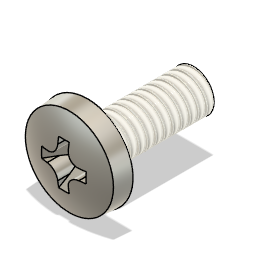
5e5ee204-5b50-4668-98c5-09c78f3fccee (Autodesk Fusion 360 design; units mm, degrees)
description: Parafuso de cabeça abaulada JIS B 1111 - M2x5
part number: BHS JIS B 1111 - M2x5 Aço 4.6 Liso
Autodesk Fusion 360 part; units mm, degrees
sketch "Sketch1" plane through (0, 0, 0) normal (0, 1, 0) x (1, 0, 0)
  line L0 (0, -1.2) -> (0, 5)
  line L1 (-2.15, 0) -> (-2.0756, -0.85)
  line L2 (-2.15, 0) -> (-0.8392, 0)
  arc A0 (-2.0756, -0.85) -> (0, -1.2) centre (0, 5.1297) ccw
  line L3 (0, 5) -> (-1, 5)
  line L4 (-1, 5) -> (-1, 0.75)
  line L5 (-1, 0.75) -> (-0.8392, 0.15)
  line L6 (-0.8392, 0.15) -> (-0.8392, 0)
  dimension "d13" = 5
  dimension "d14" = 4.3
  dimension "d18" = 2
  dimension "d23" = 15
  dimension "d53" = 1.2
  dimension "d55" = 4.25
  dimension "d56" = 5
  dimension "d57" = 4.85
  dimension "d60" = 0.85
  constraint vertical L0
  constraint coincident origin L0
  constraint horizontal L2
  constraint coincident origin L2
  constraint coincident L0 A0.end
  constraint coincident L0 A0.centre
  constraint coincident L0.start A0.end
  constraint perpendicular L0 L3
  constraint perpendicular L3 L4
  constraint vertical L6
  constraint coincident L2.end L6.end
  measures "d13" angle of L0 L1
  measures "d23" angle of L4 L5
  measures "d53" distance of L0.start L2
  measures "d55" distance of L3 L4.end
  measures "d56" distance of L2 L3
  measures "d57" distance of L3 L5.end
  measures "d60" distance of L1.end L2
revolve "Revolve1" add sketch "Sketch1" angle 360 about axis through (0, 0, 1.2) along (0, 0, -1) makes body 1
fillet "Fillet2" radius 0.1 1 edges at (-0.7824, 0.3035, 0) on bodies 1
ref_plane "WorkPlane1" through (0, 0, 1.2) normal (0, 0, 1) x (1, 0, 0)
sketch "Sketch2" plane through (0, 0, 1.2) normal (0, 0, 1) x (1, 0, 0)
  line L0 (-1.1, 0) -> (1.1, 0) construction
  line L1 (0, -1.1) -> (0, 1.1) construction
  line L2 (-0.248, 1.1) -> (0.248, 1.1)
  line L3 (0.248, 1.1) -> (0.248, 0.248)
  line L4 (0.248, 0.248) -> (1.1, 0.248)
  line L5 (1.1, 0.248) -> (1.1, -0.248)
  line L6 (1.1, -0.248) -> (0.248, -0.248)
  line L7 (0.248, -0.248) -> (0.248, -1.1)
  line L8 (0.248, -1.1) -> (-0.248, -1.1)
  line L9 (-0.248, -1.1) -> (-0.248, -0.248)
  line L10 (-0.248, -0.248) -> (-1.1, -0.248)
  line L11 (-1.1, -0.248) -> (-1.1, 0.248)
  line L12 (-1.1, 0.248) -> (-0.248, 0.248)
  line L13 (-0.248, 0.248) -> (-0.248, 1.1)
  dimension "d58" = 0.496
  dimension "d59" = 0.496
  dimension "d61" = 2.2
  dimension "d62" = 2.2
  constraint horizontal L0
  constraint vertical L1
  constraint midpoint L0 L1
  constraint midpoint origin L1
  constraint perpendicular L1 L2
  constraint perpendicular L2 L3
  constraint perpendicular L3 L4
  constraint perpendicular L0 L5
  constraint perpendicular L5 L6
  constraint perpendicular L0 L7
  constraint perpendicular L7 L8
  constraint perpendicular L8 L9
  constraint perpendicular L7 L10
  constraint perpendicular L10 L11
  constraint perpendicular L11 L12
  constraint vertical L13
  constraint coincident L9 L12.end
  constraint coincident L3.end L7
  constraint coincident L6 L9.end
  constraint coincident L4 L12.end
  constraint midpoint L0.end L5
  constraint midpoint L1.start L8
  constraint midpoint L1.end L2
  constraint midpoint L0.start L11
  measures "d58" distance of L10 L12
  measures "d59" distance of L3 L13
  measures "d61" distance of L2 L8
  measures "d62" distance of L5 L11
extrude "Extrude1" add sketch "Sketch2" against normal blind 1.01 separate body makes body 2
draft "Draft1" angle -30 neutral plane through (0, 0, 1.2) pull (0, 0, 1) 4 faces at (0.0827, -1.1, 0.8633) (-0.0827, 1.1, 0.8633) (-1.1, -0.0827, 0.8633) (1.1, 0.0827, 0.8633) on bodies 2
fillet "Fillet1" radius 0.496 4 edges at (0.248, -0.248, 0.695) (-0.248, -0.248, 0.695) (-0.248, 0.248, 0.695) (0.248, 0.248, 0.695) on bodies 2
combine "Combine1" operation cut target body 1 tool bodies 2
thread "Thread1" "ISO Metric profile 2.0 M2x0.4 M2x0.4 6g" major diameter 1.9335 minor diameter 1.478 pitch 0.4 angle 60 resizes the face on face at (-0.9988, -0.0498, -3.5833) on bodies 1
equation "adsk_nomdia = 2.00 mm"
equation "adsk_nomlen = 5.00 mm"
equation "adsk_headdia = 4.30 mm"
equation "adsk_baseh = 0.85 mm"
equation "adsk_phildia = 2.20 mm"
equation "adsk_midfillet = 0.10 mm"
equation "adsk_thrlen = 4.25 mm"
equation "adsk_phildepth = 1.01 mm"
equation "adsk_thrrun = 0.60 mm"
equation "adsk_thrang = 15.00 deg"
equation "adsk_headang = 5.00 deg"
equation "d13 = adsk_headang"
equation "d14 = adsk_headdia"
equation "adsk_ovalh = 0.35 mm"
equation "d18 = adsk_nomdia"
equation "d23 = adsk_thrang"
equation "d32 = adsk_baseh + adsk_ovalh"
equation "adsk_philwidth = 0.496 mm"
equation "d43 = -adsk_phildepth"
equation "d48 = adsk_philwidth"
equation "d52 = adsk_midfillet"
equation "d53 = adsk_baseh + adsk_ovalh"
equation "d55 = adsk_thrlen"
equation "d56 = adsk_nomlen"
equation "d57 = adsk_thrlen + adsk_thrrun"
equation "d58 = adsk_philwidth"
equation "d59 = adsk_philwidth"
equation "d60 = adsk_baseh"
equation "d61 = adsk_phildia"
equation "d62 = adsk_phildia"
